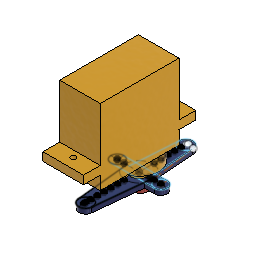
RoboarmTutorial v1 (Autodesk Fusion 360 archive; units mm, degrees)
design "MiniServo"
Autodesk Fusion 360 part; units mm, degrees
box "Grundkörper Quader1" add length 23.5 width 12.1 height 22.5 placed x (0, 1, 0) y (-1, 0, 0) z (0, 0, 1) at (2.1, 130, 14) makes body 1
sketch "Skizze2" plane through (0, 0, 14) normal (0, 0, -1) x (1, 0, 0)
  line L0 (-10, -153.5) -> (2.1, -153.5)
  line L1 (2.1, -153.5) -> (2.1, -130)
  line L2 (2.1, -130) -> (-10, -130)
  line L3 (-10, -130) -> (-10, -153.5)
  circle A0 centre (-3.95, -147.65) radius 5.85
  circle A1 centre (-3.95, -141.5) radius 2.5
  line L4 (-7.5, -141.8) -> (3, -141.8)
  line L5 (-3.95, -147.65) -> (-3.95, -135)
  circle A2 centre (-3.95, -147.65) radius 2.5
  line L6 (-10, -130) -> (2.1, -130)
  line L7 (2.1, -130) -> (2.1, -125)
  line L8 (2.1, -125) -> (-10, -125)
  line L9 (-10, -125) -> (-10, -130)
  circle A3 centre (-3.95, -128.05) radius 0.75
  line L10 (-10, -141.75) -> (-13, -141.75) construction
  circle A4 centre (-3.95, -155.45) radius 0.75
  line L11 (2.1, -158.5) -> (-10, -158.5)
  line L12 (2.1, -153.5) -> (2.1, -158.5)
  line L13 (-10, -158.5) -> (-10, -153.5)
  line L14 (-10, -153.5) -> (2.1, -153.5)
  dimension "d101" = 11.7
  dimension "d102" = 5
  dimension "d106" = 5
  dimension "d15" = 5
  dimension "d16" = 1.5
  dimension "d47" = 12
  dimension "d48" = 6.05
  dimension "d49" = 12.1
  dimension "d50" = 6.05
  dimension "d51" = 27.4
  constraint tangent L0 A0
  constraint horizontal L4
  constraint tangent A0 L4
  constraint coincident A0.centre L5.start
  constraint perpendicular L4 L5
  constraint coincident A1.centre L5
  constraint concentric A0 A2
  constraint horizontal L6
  constraint vertical L7
  constraint horizontal L8
  constraint vertical L9
  constraint coincident L2.end L3.start
  constraint coincident L1 L2.start
  constraint midpoint L3 L10.start
  constraint perpendicular L3 L10
  constraint symmetric L2.end L10 L0.start
  constraint symmetric L1.end L10 L0.end
  constraint symmetric L7.end L10 L11.start
  constraint symmetric L8.end L10 L11.end
  constraint symmetric A3 L10 A4
  measures "d101" diameter of A0
  measures "d102" diameter of A1
  measures "d106" diameter of A2
  measures "d15" distance of L2.end L8.end
  measures "d16" diameter of A3
  measures "d47" distance of A1.centre L14
  measures "d48" distance of L3 A0.centre
  measures "d49" distance of L11.start L11.end
  measures "d50" distance of A4.centre L13
  measures "d51" distance of A3.centre A4.centre
extrude "Extrusion1" add sketch "Skizze2" along normal blind 4 contours A0 A1 | A0 A1 L4 | A0 A1 L5 | A0 A1 L4 | A1 L4 L5 | A0 A1 L5 | A1 L4 L5 | A2 bodies 1
extrude "Extrusion2" add sketch "Skizze2" along normal blind 3 from surface at 4 contours A2 bodies 1
extrude "Extrusion6" add sketch "Skizze2" against normal blind 2.5 from surface at -4 contours L0 L11 L12 L13 L14 | L2 L6 L7 L8 L9 bodies 1
move_body "Verschieben1" bodies 1 to x (1, 0, 0) y (0, 1, 0) z (0, 0, 1) at (0, -3, 0)
sketch "Skizze4" plane through (0, 0, 7) normal (0, 0, -1) x (1, 0, 0)
  circle A0 centre (-3.95, -144.65) radius 2.5
  line L0 (-3.95, -126.65) -> (-3.95, -160.65) construction
  circle A1 centre (-3.95, -144.65) radius 4.1 construction
  line L1 (-12.35, -144.65) -> (4.45, -144.65) construction
  circle A2 centre (-3.9493, -158.6) radius 2.05
  circle A3 centre (-3.95, -128.7) radius 2.05
  line L2 (0.15, -144.65) -> (-1.9206, -158.8949) construction
  circle A4 centre (2.55, -144.65) radius 1.9
  circle A5 centre (-10.45, -144.65) radius 1.9
  line L3 (-10.45, -144.65) -> (-10.45, -146.55) construction
  line L4 (2.55, -144.65) -> (2.55, -146.55) construction
  line L5 (-10.45, -146.55) -> (2.55, -146.55)
  line L6 (2.55, -142.75) -> (-10.45, -142.75)
  circle A6 centre (-3.95, -140.15) radius 0.5
  circle A7 centre (-3.95, -149.15) radius 0.5
  circle A8 centre (-3.95, -138.15) radius 0.5
  circle A9 centre (-3.95, -136.15) radius 0.5
  circle A10 centre (-3.95, -151.15) radius 0.5
  circle A11 centre (-3.95, -153.15) radius 0.5
  circle A12 centre (-3.95, -134.15) radius 0.5
  circle A13 centre (-3.95, -132.15) radius 0.5
  circle A14 centre (-3.95, -130.15) radius 0.5
  circle A15 centre (-3.95, -128.15) radius 0.5
  circle A16 centre (-3.95, -155.15) radius 0.5
  circle A17 centre (-3.95, -157.15) radius 0.5
  circle A18 centre (-3.7484, -159.15) radius 0.5
  circle A19 centre (-10.45, -144.65) radius 0.5
  circle A20 centre (-8.45, -144.65) radius 0.5
  circle A21 centre (0.55, -144.65) radius 0.5
  circle A22 centre (2.55, -144.65) radius 0.5
  line L7 (-6.95, -144.65) -> (-5.9946, -158.7387)
  line L8 (-0.95, -144.65) -> (-1.9054, -158.7387)
  line L9 (-7.65, -144.65) -> (-5.9893, -128.4904)
  line L10 (-0.25, -144.65) -> (-1.9107, -128.4904)
  dimension "d4" = 34
  dimension "d5" = 8.2
  dimension "d6" = 18
  dimension "d7" = 16.8
  dimension "d8" = 4.1
  dimension "d9" = 3.8
  dimension "d28" = 1
  dimension "d29" = 1
  dimension "d30" = 9
  dimension "d31" = 4.5
  dimension "d32" = 2
  dimension "d33" = 2
  dimension "d34" = 2
  dimension "d35" = 2
  dimension "d36" = 2
  dimension "d37" = 2
  dimension "d38" = 2
  dimension "d39" = 2
  dimension "d40" = 2
  dimension "d41" = 2
  dimension "d42" = 2
  dimension "d43" = 9
  dimension "d44" = 4.5
  dimension "d45" = 2
  dimension "d46" = 2
  dimension "d53" = 0.8
  dimension "d54" = 1.5
  constraint vertical L0
  constraint coincident L0 A0.centre
  constraint horizontal L1
  constraint coincident A0.centre L1
  constraint midpoint A0.centre L1
  constraint coincident L0.end A2
  constraint coincident L0.start A3
  constraint equal A2 A3
  constraint coincident A1 L2.start
  constraint coincident L1 L2.start
  constraint coincident A2 L2.end
  constraint tangent A2 L2
  constraint coincident L1.end A4
  constraint coincident L1.start A5
  constraint equal A4 A5
  constraint coincident A5.centre L3.start
  constraint coincident A5 L3.end
  constraint perpendicular L1 L3
  constraint coincident A4.centre L4.start
  constraint coincident A4 L4.end
  constraint perpendicular L1 L4
  constraint tangent A4 L5
  constraint coincident A4 L6.start
  constraint coincident A5 L6.end
  constraint tangent A5 L6
  constraint parallel L5 L6
  constraint coincident A0.centre A1.centre
  constraint coincident L0 A6.centre
  constraint coincident L0 A7.centre
  constraint coincident L0 A8.centre
  constraint coincident L0 A9.centre
  constraint coincident L0 A10.centre
  constraint coincident L0 A11.centre
  constraint equal A6 A8
  constraint equal A6 A9
  constraint equal A6 A10
  constraint equal A6 A11
  constraint coincident L0 A12.centre
  constraint coincident L0 A13.centre
  constraint coincident L0 A14.centre
  constraint coincident L0 A15.centre
  constraint coincident L0 A16.centre
  constraint coincident L0 A17.centre
  constraint equal A9 A12
  constraint equal A12 A13
  constraint equal A12 A14
  constraint equal A12 A15
  constraint equal A11 A16
  constraint equal A11 A17
  constraint equal A11 A18
  constraint coincident L1 A5.centre
  constraint coincident L1 A20.centre
  constraint coincident L1 A21.centre
  constraint coincident L1 A4.centre
  constraint equal A6 A21
  constraint equal A6 A22
  constraint equal A6 A20
  constraint equal A6 A19
  constraint coincident L1 L7.start
  constraint coincident A2 L7.end
  constraint tangent A2 L7
  constraint symmetric L0 L7.start L8.start
  constraint symmetric L0 L7.end L8.end
  constraint coincident L1 L9.start
  constraint symmetric L0 L9.start L10.start
  constraint coincident L0 A3.centre
  constraint tangent A3 L9
  constraint tangent A3 L10
  constraint coincident A3 L10.end
  constraint coincident A3 L9.end
  measures "d4" distance of L0.start L0.end
  measures "d5" diameter of A1
  measures "d6" distance of L0.start A0.centre
  measures "d7" distance of L1.start L1.end
  measures "d8" diameter of A2
  measures "d9" diameter of A4
  measures "d28" diameter of A6
  measures "d29" diameter of A7
  measures "d30" distance of A6.centre A7.centre
  measures "d31" distance of A0.centre A7.centre
  measures "d32" distance of A6.centre A8.centre
  measures "d33" distance of A8.centre A9.centre
  measures "d34" distance of A7.centre A10.centre
  measures "d35" distance of A10.centre A11.centre
  measures "d36" distance of A9.centre A12.centre
  measures "d37" distance of A12.centre A13.centre
  measures "d38" distance of A13.centre A14.centre
  measures "d39" distance of A14.centre A15.centre
  measures "d40" distance of A11.centre A16.centre
  measures "d41" distance of A16.centre A17.centre
  measures "d42" vertical distance of A17.centre A18.centre
  measures "d43" distance of A20.centre A21.centre
  measures "d44" distance of A0.centre A21.centre
  measures "d45" distance of A5.centre A20.centre
  measures "d46" distance of A21.centre A4.centre
  measures "d53" distance of A20.centre L9.start
  measures "d54" distance of A20.centre L7.start
extrude "Extrusion4" add sketch "Skizze4" along normal blind 1.5 separate body contours A0 L5 L6 | A0 A4 L5 L6 A21 | A0 L6 | A0 A3 L6 L9 L10 | A0 A2 L5 L7 L8 | A0 L5 | A0 A5 L5 L6 A20 | A4 A21 | A3 | A2 | A5 A20 | A4 A21 | A4 A21 | A5 A20 | A5 A20 | A6 | A7 | A8 | A9 | A10 | A11 | A12 | A13 | A14 | A15 | A16 | A17 | A18 | A19 | A22 makes body 2
sketch "Skizze5" plane through (0, 0, 5.5) normal (0, 0, -1) x (1, 0, 0)
  circle A0 centre (-3.5, -144.55) radius 2.5
  line L0 (-10, -144.55) -> (3, -144.55)
  line L1 (-7.4547, -142.75) -> (-10.45, -142.75)
  arc A1 (-10.45, -142.75) -> (-10.45, -146.55) centre (-10.45, -144.65) ccw
  line L2 (-10.45, -146.55) -> (-6.8212, -146.55)
  line L3 (-6.8212, -146.55) -> (-5.9946, -158.7387)
  arc A2 (-5.9946, -158.7387) -> (-1.9003, -158.6636) centre (-3.9493, -158.6) ccw
  line L4 (-1.9003, -158.6636) -> (-1.0788, -146.55)
  line L5 (-1.0788, -146.55) -> (2.55, -146.55)
  arc A3 (2.55, -146.55) -> (2.55, -142.75) centre (2.55, -144.65) ccw
  line L6 (2.55, -142.75) -> (-0.4453, -142.75)
  line L7 (-0.4453, -142.75) -> (-1.9107, -128.4904)
  arc A4 (-1.9107, -128.4904) -> (-5.9893, -128.4904) centre (-3.95, -128.7) ccw
  line L8 (-5.9893, -128.4904) -> (-7.4547, -142.75)
  dimension "d12" = 5
  constraint coincident A0.centre L0
  constraint midpoint A0.centre L0
  measures "d12" diameter of A0
extrude "Extrusion5" add sketch "Skizze5" along normal blind 2 separate body contours A0 L0 | A0 L0 makes body 3
equation "d31 = d30 / 2"
equation "d36 = d33"
equation "d44 = d43 / 2"
equation "d45 = d34"
equation "d46 = d32"
equation "d48 = 12.10 mm / 2"
equation "d50 = d48"
